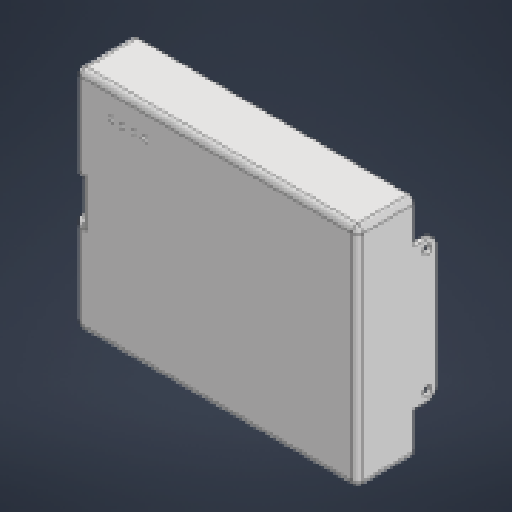
# Autodesk Inventor part: top case
Saved by Autodesk Inventor 2026.2 (Build 302298010, 298A)
## iProperties
Created: 2026-03-29
Part Number: top case
Material: 一般
Document SubType Name: Modeling
Designer: gavin
Density: 1 g/cm^3
Appearance: 預設
Author: gavin
## iProperties of the stored document top case_3D 列印.ipt
Created: 2026-03-29
Part Number: top case_3D 列印
Material: 一般
Document SubType Name: Modeling
Designer: gavin
Density: 1 g/cm^3
Appearance: 預設
Author: gavin
Autodesk Inventor part; units mm, degrees
ref_plane "YZ Plane" through (0, 0, 0) normal (1, 0, 0) x (0, 1, 0)
sketch "草圖1" plane through (0, 0, 0) normal (0, 0, 1) x (1, 0, 0)
  line L0 (4.375, 77) -> (-95.625, 77) projected
  line L1 (-95.625, 77) -> (-95.625, -3) projected
  line L2 (-95.625, -3) -> (4.375, -3) projected
  line L3 (4.375, -3) -> (4.375, 77) projected
  line L4 (-91.25, 74) -> (0, 74) projected
  line L5 (0, 0) -> (0, 74) projected
  line L6 (0, 0) -> (-91.25, 0) projected
  line L7 (-91.25, 0) -> (-91.25, 74) projected
extrude "擠出1" add sketch "草圖1" along normal blind 15.5
sketch "草圖2" plane through (0, 0, 15.5) normal (0, 0, 1) x (1, 0, 0)
  line L0 (-95.625, 77) -> (-95.625, -3) projected
  line L1 (-95.625, -3) -> (4.375, -3) projected
  line L2 (4.375, -3) -> (4.375, 77) projected
  line L3 (4.375, 77) -> (-95.625, 77) projected
  line L4 (0, 0) -> (-91.25, 0) projected
  line L5 (-91.25, 0) -> (-91.25, 74) projected
  line L6 (-91.25, 74) -> (0, 74) projected
  line L7 (0, 74) -> (0, 0) projected
extrude "擠出2" add sketch "草圖2" along normal blind 3 contours L3 L2 L1 L0 | L4 L5 L6 L7
sketch "草圖3" plane through (-95.625, -3, 0) normal (-1, 0, 0) x (0, 0, 1)
  line L0 (0, 3) -> (0, 77) projected
  line L1 (0, 77) -> (15.5, 77) projected
  line L2 (15.5, 3) -> (15.5, 77) projected
  line L3 (0, 3) -> (15.5, 3) projected
  line L4 (15.5, 77) -> (15.5, 3) projected
  line L5 (15.5, 65) -> (9.2, 65)
  line L6 (9.2, 65) -> (9.2, 15)
  line L7 (9.2, 15) -> (15.5, 15)
  line L8 (15.5, 15) -> (15.5, 65)
  point P0 (9.2, 40)
  point P1 (15.5, 40)
  point P2 (15.5, 15)
  point P3 (15.5, 65)
  dimension "d4" = 6.3
  dimension "d5" = 50
  constraints: 8 end point, 2 midpoint, 2 parallel, 1 horizontal, 1 horizontal alignment, 1 perpendicular, 1 point on line
  measures "d4" distance of L7.end L6.end
  measures "d5" distance of L6.end L5.end
extrude "擠出3" cut sketch "草圖3" against normal blind 15.5 contours L7 L6 L5 L2
ref_plane "工作平面1" through (-91.25, 4.5, 11.3) normal (0, 0, 1) x (1, 0, 0)
sketch "草圖4" plane through (0, 0, 15.5) normal (0, 0, -1) x (-1, 0, 0)
  line L0 (92.75, 4.5) -> (60.45, 4.5) construction
  line L1 (92.75, 12.38) -> (92.75, 4.5) construction
  line L2 (92.75, 12.38) -> (93.45, 12.38) construction
  line L3 (93.45, 25.41) -> (93.45, 12.38) construction
  line L4 (92.75, 25.41) -> (93.45, 25.41) construction
  line L5 (92.75, 48.59) -> (92.75, 25.41) construction
  line L6 (92.75, 48.59) -> (93.45, 48.59) construction
  line L7 (93.45, 61.62) -> (93.45, 48.59) construction
  line L8 (92.75, 61.62) -> (93.45, 61.62) construction
  line L9 (92.75, 69.5) -> (92.75, 61.62) construction
  line L10 (60.45, 69.5) -> (92.75, 69.5) construction
  line L11 (60.45, 4.5) -> (60.45, 69.5) construction
  circle A0 centre (89.75, 66.5) radius 1.5 projected
  circle A1 centre (63.45, 66.5) radius 1.5 projected
  circle A2 centre (89.75, 7.5) radius 1.5 projected
  circle A3 centre (63.45, 7.5) radius 1.5 projected
  circle A4 centre (89.75, 66.5) radius 4.165
  circle A5 centre (63.45, 66.5) radius 4.165
  circle A6 centre (63.45, 7.5) radius 4.165
  circle A7 centre (89.75, 7.5) radius 4.165
  circle A8 centre (63.45, 7.5) radius 2.165
  circle A9 centre (89.75, 7.5) radius 2.165
  circle A10 centre (89.75, 66.5) radius 2.165
  circle A11 centre (63.45, 66.5) radius 2.165
  point P0 (0, 0)
  dimension "d18" = 4.33
  dimension "d19" = 4.33
  dimension "d20" = 4.33
  dimension "d21" = 4.33
  dimension "d22" = 2
  dimension "d23" = 2
  dimension "d24" = 2
  dimension "d25" = 2
  constraints: 8 centre point, 4 coincident
  measures "d18" diameter of A8
  measures "d19" diameter of A9
  measures "d20" diameter of A10
  measures "d21" diameter of A11
  measures "d22" radial gap between concentric circles of A6 A8
  measures "d23" radial gap between concentric circles of A7 A9
  measures "d24" radial gap between concentric circles of A4 A10
  measures "d25" radial gap between concentric circles of A11 A5
extrude "擠出4" add sketch "草圖4" along normal up to surface (4.2 mm away) contours A4 | A5 | A6 | A7
sketch "草圖5" plane through (-95.625, -3, 0) normal (-1, 0, 0) x (0, 0, 1)
  line L0 (11.3, 51.59) -> (9.7, 51.59) construction
  line L1 (9.7, 51.59) -> (9.7, 28.41) construction
  line L2 (9.7, 28.41) -> (11.3, 28.41) construction
  line L3 (11.3, 37.13) -> (11.3, 28.41) construction
  arc A0 (11.3, 37.13) -> (14.5, 37.13) centre (12.9, 37.13) ccw construction
  line L4 (14.5, 37.13) -> (14.5, 42.87) construction
  arc A1 (14.5, 42.87) -> (11.3, 42.87) centre (12.9, 42.87) ccw construction
  line L5 (11.3, 51.59) -> (11.3, 42.87) construction
  line L6 (11.3, 42.87) -> (11.3, 37.13) construction
  circle A2 centre (12.9, 37.13) radius 2.6
  circle A3 centre (12.9, 42.87) radius 2.6
  line L7 (15.5, 65) -> (15.5, 15) projected
  line L8 (10.3, 42.87) -> (10.3, 37.13)
  line L9 (15.5, 65) -> (15.5, 15) projected
  line L10 (15.5, 15) -> (9.2, 15) projected
  line L11 (9.2, 15) -> (9.2, 65) projected
  line L12 (9.2, 65) -> (15.5, 65) projected
  line L13 (0, 80) -> (0, 0) projected
  line L14 (0, 0) -> (18.5, 0) projected
  line L15 (18.5, 80) -> (18.5, 0) projected
  line L16 (0, 80) -> (18.5, 80) projected
  line L17 (9.7, 51.59) -> (15.4, 51.59) projected
  line L18 (15.4, 28.41) -> (9.7, 28.41) projected
  line L19 (15.5, 51.21) -> (9.2, 51.21)
  line L20 (15.5, 28.79) -> (9.2, 28.79)
  point P0 (0, 3)
  point P1 (15.5, 37.13)
  point P2 (15.5, 42.87)
  dimension "d14" = 0.38
  dimension "d15" = 0.38
  constraints: 8 end point, 4 point on line, 3 vertical, 2 coincident, 1 collinear, 1 parallel, 1 perpendicular, 1 tangent, 6 other
  measures "d14" distance between parallel lines of L17 L19
  measures "d15" distance between parallel lines of L18 L20
extrude "擠出5" add sketch "草圖5" against normal up to surface (4.375 mm away) contours L7 L20 L11 L19 A3 L8 A2
sketch "草圖6" plane through (0, 0, 0) normal (0, 0, -1) x (-1, 0, 0)
  line L0 (95.625, 77) -> (95.625, -3) projected
  line L1 (-4.375, 77) -> (95.625, 77) projected
  line L2 (-4.375, -3) -> (-4.375, 77) projected
  line L3 (95.625, -3) -> (-4.375, -3) projected
  line L4 (0, 0) -> (91.25, 0) projected
  line L5 (0, 74) -> (0, 0) projected
  line L6 (91.25, 74) -> (0, 74) projected
  line L7 (91.25, 0) -> (91.25, 74) projected
  line L8 (-2.875, 75.5) -> (94.125, 75.5)
  line L9 (94.125, 75.5) -> (94.125, -1.5)
  line L10 (94.125, -1.5) -> (-2.875, -1.5)
  line L11 (-2.875, -1.5) -> (-2.875, 75.5)
  dimension "d26" = 1.5
  constraints: 8 end point, 3 other
  measures "d26" distance between parallel lines of L2 L11
extrude "擠出6" add sketch "草圖6" along normal blind 1.5 contours L0 L3 L2 L1
sketch "草圖7" plane through (-95.625, -3, 18.5) normal (-1, 0, 0) x (0, 0, 1)
  line L0 (-9.3, 51.21) -> (-9.3, 65) projected
  line L1 (-9.3, 65) -> (-3, 65) projected
  line L2 (-3, 65) -> (-3, 51.21) projected
  line L3 (-3, 51.21) -> (-9.3, 51.21) projected
  line L4 (-9.3, 28.79) -> (-3, 28.79) projected
  line L5 (-3, 28.79) -> (-3, 15) projected
  line L6 (-3, 15) -> (-9.3, 15) projected
  line L7 (-9.3, 15) -> (-9.3, 28.79) projected
  arc A0 (-8.2, 37.13) -> (-3, 37.13) centre (-5.6, 37.13) ccw projected
  line L8 (-8.2, 37.13) -> (-8.2, 42.87) projected
  arc A1 (-3, 42.87) -> (-8.2, 42.87) centre (-5.6, 42.87) ccw projected
  line L9 (-3, 42.87) -> (-3, 37.13) projected
  line L10 (-20, 0) -> (0, 0) projected
  line L11 (0, 80) -> (0, 0) projected
  line L12 (0, 80) -> (-20, 80) projected
  line L13 (-20, 0) -> (-20, 80) projected
  line L14 (-20, 65) -> (-24.7, 65)
  line L15 (-28, 61.7) -> (-28, 18.3)
  line L16 (-24.7, 15) -> (-20, 15)
  line L17 (-20, 15) -> (-20, 65)
  circle A2 centre (-24.7, 61.7) radius 1.65
  circle A3 centre (-24.7, 18.3) radius 1.65
  arc A4 (-24.7, 65) -> (-28, 61.7) centre (-24.7, 61.7) ccw
  arc A5 (-28, 18.3) -> (-24.7, 15) centre (-24.7, 18.3) ccw
  point P0 (-18.5, 3)
  point P1 (-28, 15)
  point P2 (-28, 65)
  point P3 (-28, 40)
  point P4 (-20, 40)
  dimension "d29" = 8
  dimension "d30" = 50
  dimension "d31" = 3.3
  dimension "d32" = 3.3
  dimension "d33" = 3.3
  dimension "d34" = 3.3
  dimension "d35" = 3.3
  dimension "d36" = 3.3
  dimension "d37" = 3.3
  constraints: 8 end point, 5 point on line, 4 centre point, 4 point on circle, 4 tangent, 2 midpoint, 2 parallel, 1 equal radius, 1 horizontal, 1 horizontal alignment, 1 perpendicular
  measures "d29" distance of L16.end point (-28, 15)
  measures "d30" distance of point (-28, 65) point (-28, 15)
  measures "d31" diameter of A2
  measures "d32" diameter of A3
  measures "d33" distance from line of L14 A2.centre
  measures "d34" distance from line of L15 A2.centre
  measures "d35" distance from line of L15 A3.centre
  measures "d36" distance from line of L16 A3.centre
  measures "d37" radius of A4
extrude "擠出7" add sketch "草圖7" against normal blind 1.5 contours L16 A5 L15 A4 L14 L13
ref_plane "工作平面2" through (-45.625, -3, 18.5) normal (-1, 0, 0) x (0, 0, 1)
mirror "鏡射1" about plane through (-45.625, -3, 18.5) normal (-1, 0, 0) of "擠出7"
sketch "草圖9" plane through (-91.25, 0, 0) normal (0, 1, 0) x (1, 0, 0)
  circle A0 centre (8.35, -12.89) radius 0.95 projected
  line L0 (10.35, -14.89) -> (6.35, -14.89)
  line L1 (6.35, -14.89) -> (6.35, -10.89)
  line L2 (6.35, -10.89) -> (10.35, -10.89)
  line L3 (10.35, -10.89) -> (10.35, -14.89)
  line L4 (10.35, -14.89) -> (6.35, -10.89) construction
  line L5 (6.35, -14.89) -> (10.35, -10.89) construction
  line L6 (10.35, -10.89) -> (21.35, -10.89)
  line L7 (21.35, -10.89) -> (21.35, -14.89)
  line L8 (21.35, -14.89) -> (10.35, -14.89)
  line L9 (10.35, -14.89) -> (10.35, -10.89)
  circle A1 centre (8.35, -12.89) radius 0.95 projected
  line L10 (10.35, -14.89) -> (6.35, -14.89)
  line L11 (6.35, -14.89) -> (6.35, -10.89)
  line L12 (6.35, -10.89) -> (10.35, -10.89)
  line L13 (10.35, -10.89) -> (10.35, -14.89)
  line L14 (10.35, -14.89) -> (6.35, -10.89) construction
  line L15 (6.35, -14.89) -> (10.35, -10.89) construction
  point P0 (91.25, 0)
  dimension "d43" = 4
  dimension "d44" = 4
  dimension "d45" = 11
  dimension "d46" = 4
  dimension "d78" = 4
  constraints: 32 end point, 6 parallel, 4 midpoint, 3 horizontal, 3 perpendicular
  measures "d43" distance of L1.end L2.end
  measures "d44" distance of L0.end L1.end
  measures "d45" distance of L7.end L8.end
  measures "d46" distance of L6.end L7.end
  measures "d78" distance of L11.end L12.end
extrude "擠出9" cut sketch "草圖9" against normal through all contours A0 | L0 L1 L2 L3 | L3 L6 L7 L8
fillet "圓角2" radius 2 7 edges at (-95.625, 77, 8.5) (-45.625, 77, 18.5) (-95.625, -3, 8.5) (-45.625, -3, 18.5) (4.375, 37, 18.5) (4.375, -3, 8.5) (4.375, 77, 8.5)
sketch "草圖13" plane through (0, 0, 0) normal (0, 0, -1) x (-1, 0, 0)
  line L0 (-2.875, 75.5) -> (-2.875, -1.5) projected
  line L1 (-2.875, -1.5) -> (94.125, -1.5) projected
  line L2 (94.125, -1.5) -> (94.125, 75.5) projected
  line L3 (94.125, 75.5) -> (-2.875, 75.5) projected
  line L4 (0, 0) -> (91.25, 0) projected
  line L5 (0, 74) -> (0, 0) projected
  line L6 (91.25, 74) -> (0, 74) projected
  line L7 (91.25, 0) -> (91.25, 74) projected
  arc A0 (91.25, 68.0612) -> (91.25, 64.9388) centre (89.75, 66.5) ccw projected
  arc A1 (91.25, 9.0612) -> (91.25, 5.9388) centre (89.75, 7.5) ccw projected
  line L8 (91.25, 74) -> (92.75, 74)
  line L9 (92.75, 74) -> (92.75, 0)
  line L10 (92.75, 0) -> (91.25, 0)
  line L11 (91.25, 0) -> (91.25, 74)
  dimension "d58" = 1.5
  constraints: 8 end point, 2 parallel, 1 horizontal, 1 perpendicular
  measures "d58" distance of L9.end L10.end
extrude "擠出12" cut sketch "草圖13" against normal up to surface (15.5 mm away) contours L7 L8 L9 L10
sketch "草圖14" plane through (-89.75, 66.5, 11.3) normal (0, 0, -1) x (-1, 0, 0)
  line L0 (1.5, 3.8855) -> (1.5, 1.5612) projected
  arc A0 (1.5, 3.8855) -> (1.5, -3.8855) centre (0, 0) ccw projected
  line L1 (1.5, -1.5612) -> (1.5, -3.8855) projected
  arc A1 (1.5, 1.5612) -> (1.5, -1.5612) centre (0, 0) ccw projected
  line L2 (1.5, -60.5612) -> (1.5, -62.8855) projected
  arc A2 (1.5, -57.4388) -> (1.5, -60.5612) centre (0, -59) ccw projected
  line L3 (1.5, -55.1145) -> (1.5, -57.4388) projected
  arc A3 (1.5, -55.1145) -> (1.5, -62.8855) centre (0, -59) ccw projected
  circle A4 centre (0, -59) radius 2.165
  circle A5 centre (0, -59) radius 4.165
  circle A6 centre (0, 0) radius 2.165
  circle A7 centre (0, 0) radius 4.165
  point P0 (-89.75, -66.5)
  constraints: 4 coincident, 12 other
extrude "擠出13" add sketch "草圖14" against normal up to surface (4.2 mm away) contours A7 L1 A6 L0 | A4 L3 A5 L2
sketch "草圖15" plane through (-95.625, 15.3, -9.5) normal (-1, 0, 0) x (0, 0, 1)
  line L0 (28, -16.3) -> (8, -16.3) projected
  line L1 (28, 59.7) -> (28, -16.3) projected
  line L2 (8, 59.7) -> (28, 59.7) projected
  line L3 (8, 46.7) -> (8, 59.7) projected
  line L4 (8, 46.7) -> (3.3, 46.7) projected
  arc A0 (3.3, 46.7) -> (0, 43.4) centre (3.3, 43.4) ccw projected
  line L5 (0, 43.4) -> (0, 0) projected
  arc A1 (0, 0) -> (3.3, -3.3) centre (3.3, 0) ccw projected
  line L6 (3.3, -3.3) -> (8, -3.3) projected
  line L7 (8, -16.3) -> (8, -3.3) projected
  arc A2 (19.8, 18.83) -> (25, 18.83) centre (22.4, 18.83) ccw projected
  line L8 (19.8, 18.83) -> (19.8, 24.57) projected
  arc A3 (25, 24.57) -> (19.8, 24.57) centre (22.4, 24.57) ccw projected
  line L9 (25, 24.57) -> (25, 18.83) projected
  line L10 (18.7, 10.49) -> (25, 10.49) projected
  line L11 (25, 10.49) -> (25, -3.3) projected
  line L12 (25, -3.3) -> (18.7, -3.3) projected
  line L13 (18.7, -3.3) -> (18.7, 10.49) projected
  line L14 (18.7, 32.91) -> (18.7, 46.7) projected
  line L15 (18.7, 46.7) -> (25, 46.7) projected
  line L16 (25, 46.7) -> (25, 32.91) projected
  line L17 (25, 32.91) -> (18.7, 32.91) projected
  circle A4 centre (3.3, 0) radius 1.65 projected
  circle A5 centre (3.3, 43.4) radius 1.65 projected
  line L18 (28, 28.27) -> (18.7, 28.27)
  line L19 (18.7, 28.27) -> (18.7, 15.13)
  line L20 (18.7, 15.13) -> (28, 15.13)
  line L21 (28, 15.13) -> (28, 28.27)
  point P0 (9.5, -15.3)
  point P1 (18.7, 21.7)
  point P2 (28, 15.13)
  dimension "d63" = 1.1
  dimension "d64" = 3.7
  dimension "d65" = 2.6
  dimension "d66" = 3.7
  constraints: 8 end point, 2 parallel, 1 horizontal, 1 midpoint, 1 perpendicular, 1 point on line, 1 vertical alignment
  measures "d63" distance between parallel lines of L19 L8
  measures "d64" distance from line of L20 A2.centre
  measures "d65" radius of A2
  measures "d66" distance from line of L18 A3.centre
extrude "擠出14" cut sketch "草圖15" against normal blind 1.875 contours L20 L19 L18 L1
fillet "圓角3" radius 2 7 edges at (-95.0392, 76.4142, 17.9142) (-95.625, 59.285, 18.5) (-93.75, 37, 18.5) (-94.6875, 30.43, 18.5) (-95.0392, -2.4142, 17.9142) (-95.625, 14.715, 18.5) (-94.6875, 43.57, 18.5)
sketch "草圖16" plane through (0, 0, 18.5) normal (0, 0, 1) x (1, 0, 0)
  line L0 (-79.51, 67.7) -> (-78.51, 67.7) projected
  line L1 (-78.51, 67.7) -> (-78.51, 66.7) projected
  line L2 (-78.51, 66.7) -> (-79.51, 66.7) projected
  line L3 (-79.51, 66.7) -> (-79.51, 67.7) projected
  line L4 (-75.51, 66.7) -> (-75.51, 67.7) projected
  line L5 (-75.51, 67.7) -> (-74.51, 67.7) projected
  line L6 (-74.51, 67.7) -> (-74.51, 66.7) projected
  line L7 (-74.51, 66.7) -> (-75.51, 66.7) projected
  line L8 (-83.51, 67.7) -> (-82.51, 67.7) projected
  line L9 (-82.51, 67.7) -> (-82.51, 66.7) projected
  line L10 (-82.51, 66.7) -> (-83.51, 66.7) projected
  line L11 (-83.51, 66.7) -> (-83.51, 67.7) projected
  line L12 (-71.51, 67.7) -> (-70.51, 67.7) projected
  line L13 (-70.51, 67.7) -> (-70.51, 66.7) projected
  line L14 (-70.51, 66.7) -> (-71.51, 66.7) projected
  line L15 (-71.51, 66.7) -> (-71.51, 67.7) projected
  circle A0 centre (-63.45, 7.5) radius 1.5 projected
  circle A1 centre (-89.75, 7.5) radius 1.5 projected
  circle A2 centre (-63.45, 66.5) radius 1.5 projected
  circle A3 centre (-89.75, 66.5) radius 1.5 projected
  line L16 (-85.25, 4.5) -> (-85.25, 7.9) projected
  line L17 (-85.25, 7.9) -> (-80.55, 7.9) projected
  line L18 (-80.55, 7.9) -> (-80.55, 4.5) projected
  line L19 (-80.55, 4.5) -> (-60.45, 4.5) projected
  line L20 (-60.45, 4.5) -> (-60.45, 69.5) projected
  line L21 (-60.45, 69.5) -> (-92.75, 69.5) projected
  line L22 (-92.75, 69.5) -> (-92.75, 61.62) projected
  line L23 (-92.75, 61.62) -> (-82.65, 61.62) projected
  line L24 (-82.65, 61.62) -> (-82.65, 48.59) projected
  line L25 (-82.65, 48.59) -> (-92.75, 48.59) projected
  line L26 (-92.75, 48.59) -> (-92.75, 39.87) projected
  line L27 (-92.75, 39.87) -> (-85.35, 39.87) projected
  line L28 (-85.35, 39.87) -> (-85.35, 34.13) projected
  line L29 (-92.75, 34.13) -> (-85.35, 34.13) projected
  line L30 (-92.75, 34.13) -> (-92.75, 25.41) projected
  line L31 (-92.75, 25.41) -> (-82.65, 25.41) projected
  line L32 (-82.65, 25.41) -> (-82.65, 12.38) projected
  line L33 (-82.65, 12.38) -> (-92.75, 12.38) projected
  line L34 (-92.75, 12.38) -> (-92.75, 4.5) projected
  line L35 (-92.75, 4.5) -> (-85.25, 4.5) projected
  circle A4 centre (-71.01, 67.2) radius 1
  circle A5 centre (-75.01, 67.2) radius 1
  circle A6 centre (-79.01, 67.2) radius 1
  circle A7 centre (-83.01, 67.2) radius 1
  point P0 (0, 0)
  dimension "d70" = 2
  dimension "d71" = 2
  dimension "d72" = 2
  dimension "d73" = 2
  constraints: 4 centre point
  measures "d70" diameter of A4
  measures "d71" diameter of A5
  measures "d72" diameter of A6
  measures "d73" diameter of A7
extrude "擠出15" cut sketch "草圖16" against normal up to surface (3 mm away) contours L0 L1 L2 L3 | L4 L5 L6 L7 | L8 L9 L10 L11 | L12 L13 L14 L15 | A4 | A5 | A6 | A7
sketch "草圖17" plane through (0, 0, 15.5) normal (0, 0, -1) x (-1, 0, 0)
  circle A0 centre (63.45, 66.5) radius 2.165 projected
  circle A1 centre (89.75, 66.5) radius 1.5 projected
  circle A2 centre (89.75, 66.5) radius 2.165 projected
  circle A3 centre (63.45, 7.5) radius 2.165 projected
  circle A4 centre (89.75, 7.5) radius 2.165 projected
  point P0 (0, 0)
extrude "擠出16" cut sketch "草圖17" against normal blind 1.5 contours A0 | A1 | A2 | A3 | A4
equation "\"d34\" = d33"
equation "\"d35\" = d34"
equation "\"d36\" = d33"
equation "\"d64\" = d65 + d63"
equation "\"d66\" = d64"
